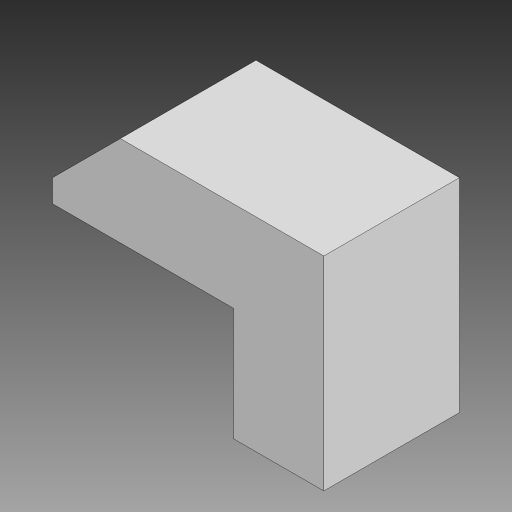
# Autodesk Inventor part: sonar-liner
Saved by Autodesk Inventor 2023 (Build 270158000, 158)
## iProperties
Created: 2024-02-27
Part Number: sonar-liner
Material: Všeobecné
Document SubType Name: Modeling
Designer: mates.exe
Mass: 0.047625 g
Surface Area: 0.92114 cm^2
Volume: 0.047625 cm^3
Density: 1 g/cm^3
Appearance: Výchozí
Author: mates.exe
## iProperties of the stored document sonar-liner_3D tisk.ipt
Created: 2024-02-27
Part Number: sonar-liner_3D tisk
Material: Všeobecné
Document SubType Name: Modeling
Designer: mates.exe
Mass: 0.047625 g
Surface Area: 0.92114 cm^2
Volume: 0.047625 cm^3
Density: 1 g/cm^3
Appearance: Výchozí
Author: mates.exe
Autodesk Inventor part; units mm, degrees
ref_plane "YZ Plane" through (0, 0, 0) normal (1, 0, 0) x (0, 1, 0)
ref_plane "XZ Plane" through (0, 0, 0) normal (0, 1, 0) x (-1, 0, 0)
ref_plane "XY Plane" through (0, 0, 0) normal (0, 0, 1) x (1, 0, 0)
sketch "Náčrt1" plane through (0, 0, 0) normal (0, 0, 1) x (1, 0, 0)
  line L0 (-3, -1) -> (3, -1)
  line L1 (3, -1) -> (3, 1)
  line L2 (3, 1) -> (-3, 1)
  line L3 (-3, 1) -> (-3, -1)
  line L4 (-3, -1) -> (3, 1) construction
  line L5 (3, -1) -> (-3, 1) construction
  line L6 (3, 1) -> (1, 1)
  line L7 (1, 1) -> (1, -3.5)
  line L8 (1, -3.5) -> (3, -3.5)
  line L9 (3, -3.5) -> (3, 1)
  point P0 (0, 0)
  point P1 (1, -1)
  dimension "d0" = 6
  dimension "d1" = 2
  dimension "d2" = 2
  dimension "d3" = 4.5
  constraints: 20 end point, 4 parallel, 2 horizontal, 2 midpoint, 2 perpendicular
  measures "d0" distance of L2.end L1.end
  measures "d1" distance of L1.end L0.end
  measures "d2" distance of L8.end L7.end
  measures "d3" distance of L7.end L6.end
extrude "Vysunutí1" add sketch "Náčrt1" along normal blind 3
chamfer "Zkosení1" distance 1.5 angle 45 1 edges at (-3, 1, 1.5)
